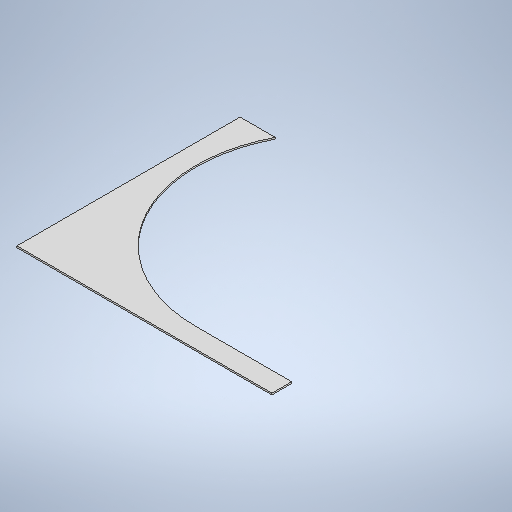
# Autodesk Inventor part: WoodBoundaryV1
Saved by Autodesk Inventor 2025.1 (Build 291241000, 241)
## iProperties
Created: 2025-10-12
Part Number: WoodBoundaryV1
Material: Generic
Document SubType Name: Modeling
Designer: jonas
Density: 1 g/cm^3
Appearance: Default
Author: jonas
Autodesk Inventor part; units mm, degrees
ref_plane "YZ Plane" through (0, 0, 0) normal (1, 0, 0) x (0, 1, 0)
ref_plane "XZ Plane" through (0, 0, 0) normal (0, 1, 0) x (-1, 0, 0)
ref_plane "XY Plane" through (0, 0, 0) normal (0, 0, 1) x (1, 0, 0)
sketch "Sketch1" plane through (0, 0, 0) normal (0, 1, 0) x (-1, 0, 0)
  line L0 (0, -151.455) -> (0, 151.455) construction
  line L1 (30.6851, 0) -> (-30.6851, 0) construction
  arc A0 (389.7841, -200) -> (0, 438.1) centre (0, 0) ccw
  line L2 (0, 438.1) -> (-300, 438.1)
  line L3 (-300, 438.1) -> (-300, 500)
  line L4 (-300, 500) -> (500, 500)
  line L5 (500, 500) -> (500, -200)
  line L6 (500, -200) -> (389.7841, -200)
  dimension "d0" = 876.2
  dimension "d8" = 500
  dimension "d9" = 500
  dimension "d10" = 700
  dimension "d11" = 300
  constraints: 14 end point, 3 perpendicular, 2 coincident, 2 horizontal, 2 midpoint, 2 point on circle, 2 vertical, 1 centre point, 1 tangent
  measures "d0" diameter of A0
  measures "d8" distance between parallel lines of L0 L5
  measures "d9" distance between parallel lines of L4 L1
  measures "d10" distance between parallel lines of L4 L6
  measures "d11" distance between parallel lines of L0 L3
extrude "Extrusion1" add sketch "Sketch1" along normal blind 5
body "Solid1"
